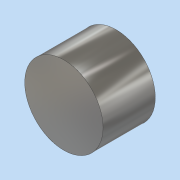
# Autodesk Inventor part: EncoderMagnet
Saved by Autodesk Inventor 2017 (Build 210142000, 142)
## iProperties
Created: 2018-04-11
Part Number: EncoderMagnet
Material: Nickel-Copper Alloy 400
Document SubType Name: Modeling
Designer: Derek Wider
Density: 8.83 g/cm^3
Appearance: Chrome - Polished
Author: Derek Wider
Autodesk Inventor part; units mm, degrees
ref_plane "YZ Plane" through (0, 0, 0) normal (1, 0, 0) x (0, 1, 0)
ref_plane "XZ Plane" through (0, 0, 0) normal (0, 1, 0) x (-1, 0, 0)
ref_plane "XY Plane" through (0, 0, 0) normal (0, 0, 1) x (1, 0, 0)
sketch "Sketch2" plane through (0, 0, 0) normal (0, 0, 1) x (1, 0, 0)
  circle A0 centre (0, 0) radius 1.5
  dimension "d0" = 3
  constraints: 1 centre point, 1 coincident
  measures "d0" diameter of A0
extrude "Extrusion1" add sketch "Sketch2" along normal blind 2
body "Solid1"
